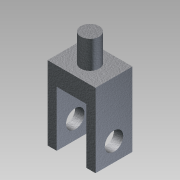
# Autodesk Inventor part: small wheel support
Saved by Autodesk Inventor 2012 (Build 160160000, 160)
## iProperties
Created: 2012-09-15
Part Number: small wheel support
Material: Default
Document SubType Name: Modeling
Designer: Admin
Density: 1 g/cm^3
Author: Admin
Autodesk Inventor part; units mm, degrees
ref_plane "YZ Plane" through (0, 0, 0) normal (1, 0, 0) x (0, 1, 0)
ref_plane "XZ Plane" through (0, 0, 0) normal (0, 1, 0) x (-1, 0, 0)
ref_plane "XY Plane" through (0, 0, 0) normal (0, 0, 1) x (1, 0, 0)
sketch "Sketch1" plane through (0, 0, 0) normal (0, 0, 1) x (1, 0, 0)
  line L0 (-33.02, 0) -> (-33.02, 50.8)
  line L1 (-33.02, 50.8) -> (0, 50.8)
  line L2 (0, 50.8) -> (0, 0)
  line L3 (-33.02, 0) -> (-26.67, 0)
  line L4 (-26.67, 0) -> (-26.67, 38.1)
  line L5 (-33.02, 50.8) -> (-33.02, 44.45)
  line L6 (-26.67, 38.1) -> (-6.35, 38.1)
  line L7 (0, 50.8) -> (-6.35, 50.8)
  line L8 (-6.35, 38.1) -> (-6.35, 0)
  line L9 (0, 0) -> (-6.35, 0)
  line L10 (-26.67, 0) -> (-33.02, 0)
  dimension "d0" = 33.02
  dimension "d1" = 50.8
  dimension "d2" = 6.35
  dimension "d3" = 6.35
  dimension "d4" = 6.35
  dimension "d11" = 50.8
  dimension "d15" = 38.1
  constraints: 22 end point, 6 perpendicular, 3 parallel, 2 horizontal, 2 point on line
  measures "d0" distance of L0.end L1.end
  measures "d1" distance of L1.end L2.end
  measures "d2" distance of L0.start L3.end
  measures "d3" distance of L0.end L5.end
  measures "d4" distance of L1.end L7.end
  measures "d11" distance of L0.start L0.end
  measures "d15" distance of L3.end L4.end
extrude "Extrusion1" add sketch "Sketch1" along normal blind 25.4
sketch "Sketch2" plane through (0, 0, 0) normal (1, 0, 0) x (0, 0, -1)
  line L0 (0, 0) -> (-25.4, 0) projected
  line L1 (0, 50.8) -> (-25.4, 50.8) projected
  line L2 (-12.7, 0) -> (-12.7, 12.7)
  circle A0 centre (-12.7, 12.7) radius 6.35
  dimension "d7" = 12.7
  dimension "d8" = 12.7
  constraints: 2 end point, 1 centre point, 1 coincident, 1 midpoint, 1 perpendicular
  measures "d7" distance of L2.start L2.end
  measures "d8" diameter of A0
extrude "Extrusion2" cut sketch "Sketch2" against normal blind 254
sketch "Sketch3" plane through (-33.02, 50.8, 0) normal (0, 1, 0) x (1, 0, 0)
  circle A0 centre (16.51, -12.7) radius 6.35
  dimension "d12" = 12.7
  constraints: 1 centre point
  measures "d12" diameter of A0
extrude "Extrusion3" add sketch "Sketch3" along normal blind 19.05
body "Solid1"
